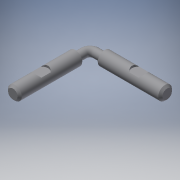
# Autodesk Inventor part: 20-128Z1
Saved by Autodesk Inventor 2018 (Build 220105000, 105)
## iProperties
Created: 2004-11-19
Part Number: 20-128Z1
Document SubType Name: Modeling
Designer: Autodesk, Inc.
Manufacturer: Standard
Standards Organization: Custom
Description: 90° MITRE CONNECTOR
Vendor: PARKER IPS
Mass: 2.13496 g
Surface Area: 14.8989 cm^2
Volume: 2.13496 cm^3
Density: 1 g/cm^3
Sheet Metal Rule: Default
Material: Generic
Appearance: Default
CAGE: 1LJX3
Dept. ID: Product Design
Description #2: ---
Finish #1: ---
Finish #2: ---
Material ID: ---
Project Number: ---
Author: Autodesk, Inc.
Autodesk Inventor part; units mm, degrees
ref_plane "YZ Plane" through (0, 0, 0) normal (1, 0, 0) x (0, 1, 0)
ref_plane "Work Plane1" through (0, 0, 7) normal (0, 0, 1) x (1, 0, 0)
sketch "Sketch1" plane through (0, 0, 7) normal (0, 0, 1) x (1, 0, 0)
  circle A0 centre (0, 0) radius 3.285
  dimension "d0" = 6.57
  constraints: 1 centre point, 1 other
  measures "d0" diameter of A0
extrude "Extrusion1" add sketch "Sketch1" along normal blind 30
chamfer "Chamfer1" distance 1 angle 45 1 edges at (-3.285, 0, 37)
ref_plane "Work Plane2" through (0, 3.285, 7) normal (0, 1, 0) x (-1, 0, 0)
sketch "Sketch2" plane through (0, 3.285, 7) normal (0, 1, 0) x (-1, 0, 0)
  line L0 (3.285, 0) -> (3.285, 29) projected
  line L1 (-3.285, 0) -> (-3.285, 29) projected
  circle A0 centre (0, 16.4) radius 3.285
  point P0 (0, -7)
  dimension "d10" = 23.4
  constraints: 2 tangent, 1 centre point
  measures "d10" distance of point (0, -7) A0.centre
extrude "Extrusion2" cut sketch "Sketch2" against normal blind 1
pattern_circular "Circular Pattern1" count 2 over 90 about axis through (0, -10, 0) along (0, 1, 0) of "Extrusion1", "Chamfer1", "Extrusion2"
sketch "Sketch3" plane through (0, 0, 0) normal (0, 1, 0) x (-1, 0, 0)
  line L0 (-7, -3.285) -> (-7, 3.285) projected
  line L1 (-3.285, 7) -> (3.285, 7) projected
  line L2 (-7, 0) -> (-3, 0)
  line L3 (0, 3) -> (0, 7)
  arc A0 (-3, 0) -> (0, 3) centre (-3, 3) ccw
  dimension "d13" = 3
  constraints: 4 end point, 2 midpoint, 2 point on circle, 2 tangent, 1 centre point, 1 parallel, 1 vertical
  measures "d13" radius of A0
sketch "Sketch4" plane through (0, 0, 7) normal (0, 0, -1) x (-1, 0, 0)
  circle A0 centre (0, 0) radius 3.285 construction
  circle A1 centre (0, 0) radius 2
  dimension "d14" = 4
  constraints: 1 centre point, 1 coincident
  measures "d14" diameter of A1
sweep "Sweep1" add profiles "Sketch4" path "Sketch3" path curves L3 A0 L2
equation "\"BendRadius\" = Thickness"
equation "\"BendReliefWidth\" = Thickness"
equation "\"BendReliefDepth\" = 0.5 * Thickness"
equation "\"CornerReliefSize\" = 4 * Thickness"
equation "\"MinimumRemnant\" = 2 * Thickness"
equation "\"TransitionRadius\" = BendRadius"
equation "\"JacobiRadiusSize\" = Thickness"
equation "\"GapSize\" = Thickness"
equation "\"Thickness\" = 3.048"
body "Solid1"
